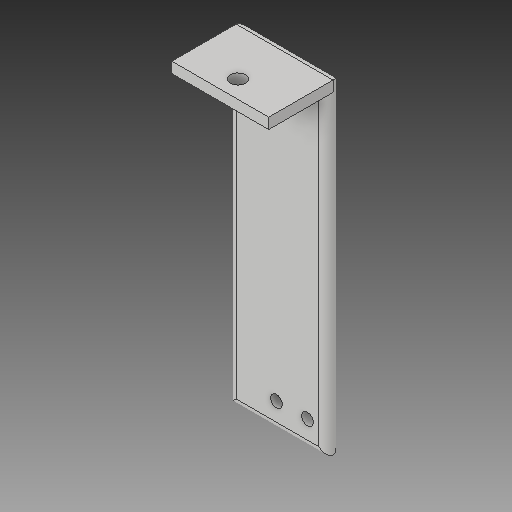
# Autodesk Inventor part: Chain_fixture
Saved by Autodesk Inventor 2019.3 (Build 233278000, 278)
## iProperties
Created: 2020-09-10
Part Number: Chain_fixture
Material: Generisch
Document SubType Name: Modeling
Designer: Nicolas Frick
Density: 1 g/cm^3
Appearance: Vorgabe
Author: Nicolas Frick
Autodesk Inventor part; units mm, degrees
ref_plane "YZ Plane" through (0, 0, 0) normal (1, 0, 0) x (0, 1, 0)
ref_plane "XZ Plane" through (0, 0, 0) normal (0, 1, 0) x (-1, 0, 0)
ref_plane "XY Plane" through (0, 0, 0) normal (0, 0, 1) x (1, 0, 0)
sketch "Skizze1" plane through (0, 0, 0) normal (0, 0, 1) x (1, 0, 0)
  line L0 (10, 15) -> (45.7133, 15) construction
  line L1 (10, 15) -> (10, -10) construction
  line L2 (37.1394, -10) -> (10, -10) construction
  line L3 (37.1394, -10) -> (37.1394, 14.1) construction
  line L4 (37.1394, 14.1) -> (45.7133, 14.1) construction
  line L5 (45.7133, 14.1) -> (45.7133, 15) construction
  line L6 (10, -10) -> (37.1394, -10)
  line L7 (37.1394, -10) -> (37.1394, 59.9176)
  line L8 (37.1394, 59.9176) -> (10, 59.9176)
  line L9 (10, 59.9176) -> (10, -10)
  point P0 (0, 0)
  constraints: 8 end point, 2 parallel, 1 horizontal, 1 perpendicular
extrude "Extrusion1" add sketch "Skizze1" along normal blind 4
sketch "Skizze2" plane through (0, 0, 0) normal (0, 0, -1) x (-1, 0, 0)
  line L0 (-37.1394, 59.9176) -> (-10, 59.9176) projected
  line L1 (-10, 59.9176) -> (-37.1394, 59.9176)
  line L2 (-37.1394, 59.9176) -> (-37.1394, 62.9176)
  line L3 (-37.1394, 62.9176) -> (-10, 62.9176)
  line L4 (-10, 62.9176) -> (-10, 59.9176)
  point P0 (0, 0)
  dimension "d2" = 3
  constraints: 8 end point, 2 parallel, 1 horizontal, 1 perpendicular
  measures "d2" distance of L1.end L2.end
extrude "Extrusion2" add sketch "Skizze2" against normal blind 20
sketch "Skizze4" plane through (10, 62.9176, 0) normal (0, 1, 0) x (1, 0, 0)
  line L0 (27.1394, -4) -> (27.1394, -73.6709) construction
  line L1 (-71.0464, -73.5081) -> (53.1741, -73.5081) construction
  line L2 (53.1741, -72.4315) -> (53.1741, -73.5081) construction
  arc A0 (58.1741, -67.4315) -> (53.1741, -72.4315) centre (58.1741, -72.4315) ccw construction
  line L3 (62.2394, -67.4315) -> (58.1741, -67.4315) construction
  line L4 (62.2394, -59.1955) -> (62.2394, -67.4315) construction
  arc A1 (65.5394, -59.1955) -> (62.2394, -59.1955) centre (63.8894, -59.1955) ccw construction
  line L5 (65.5394, -67.4315) -> (65.5394, -59.1955) construction
  line L6 (81.2394, -67.4315) -> (65.5394, -67.4315) construction
  arc A2 (76.4341, -48.82) -> (81.2394, -67.4315) centre (125.2788, -46.1349) ccw construction
  arc A3 (76.4267, -48.4999) -> (76.4341, -48.82) centre (81.4265, -48.5455) ccw construction
  arc A4 (76.4267, -48.4999) -> (35.4184, -9) centre (29.7163, -55.9569) ccw construction
  line L7 (35.4184, -9) -> (-5, -9) construction
  line L8 (-5, -9) -> (-5, 9.9226) construction
  line L9 (-5, 9.9226) -> (-10, 9.9226) construction
  line L10 (-10, 9.9226) -> (-10, 9.9096) construction
  line L11 (-10, 9.9096) -> (-37.7867, 9.9096) construction
  arc A5 (-37.7867, 9.9096) -> (-54.9732, -24.6463) centre (-14.5965, -23.176) ccw construction
  arc A6 (-54.9732, -24.6463) -> (-71.0464, -73.5081) centre (23.4557, -77.5201) ccw construction
  arc A7 (-40.4634, -62.3724) -> (-28.4634, -62.3724) centre (-34.4634, -62.3724) ccw construction
  line L12 (-40.4634, -62.3724) -> (-40.4634, -47.5724) construction
  arc A8 (-28.4634, -47.5724) -> (-40.4634, -47.5724) centre (-34.4634, -47.5724) ccw construction
  line L13 (-28.4634, -47.5724) -> (-28.4634, -62.3724) construction
  arc A9 (-40.4634, -16.9802) -> (-28.4634, -16.9802) centre (-34.4634, -16.9802) ccw construction
  line L14 (-40.4634, -16.9802) -> (-40.4634, -2.1802) construction
  arc A10 (-28.4634, -2.1802) -> (-40.4634, -2.1802) centre (-34.4634, -2.1802) ccw construction
  line L15 (-28.4634, -2.1802) -> (-28.4634, -16.9802) construction
  line L16 (37.2394, -63.0832) -> (59.5394, -63.0832) construction
  line L17 (37.2394, -34.3078) -> (37.2394, -63.0832) construction
  arc A11 (59.5394, -34.3078) -> (37.2394, -34.3078) centre (48.3894, -34.3078) ccw construction
  line L18 (59.5394, -63.0832) -> (59.5394, -34.3078) construction
  arc A12 (62.2394, -38.1955) -> (65.5394, -38.1955) centre (63.8894, -38.1955) ccw construction
  line L19 (62.2394, -28.1955) -> (62.2394, -38.1955) construction
  arc A13 (65.5394, -28.1955) -> (62.2394, -28.1955) centre (63.8894, -28.1955) ccw construction
  line L20 (65.5394, -38.1955) -> (65.5394, -28.1955) construction
  arc A14 (34.5394, -59.1955) -> (31.2394, -59.1955) centre (32.8894, -59.1955) ccw construction
  line L21 (34.5394, -67.4315) -> (34.5394, -59.1955) construction
  line L22 (31.2394, -67.4315) -> (34.5394, -67.4315) construction
  line L23 (31.2394, -59.1955) -> (31.2394, -67.4315) construction
  arc A15 (31.2394, -38.1955) -> (34.5394, -38.1955) centre (32.8894, -38.1955) ccw construction
  line L24 (31.2394, -28.1955) -> (31.2394, -38.1955) construction
  arc A16 (34.5394, -28.1955) -> (31.2394, -28.1955) centre (32.8894, -28.1955) ccw construction
  line L25 (34.5394, -38.1955) -> (34.5394, -28.1955) construction
  line L26 (0, -4) -> (0, -78.5081) construction
  line L27 (27.1394, -20) -> (0, -20) construction
  circle A17 centre (13.5697, -15.0495) radius 2.1
  point P0 (-10, 0)
  dimension "d11" = 4.2
  constraints: 1 centre point
  measures "d11" diameter of A17
extrude "Extrusion4" cut sketch "Skizze4" against normal through all
sketch "Skizze5" plane through (10, -10, 0) normal (0, -1, 0) x (1, 0, 0)
  line L0 (0, 0) -> (27.1394, 0) projected
  line L1 (27.1394, 0) -> (27.1394, 4) projected
  line L2 (0, 4) -> (27.1394, 4) projected
  line L3 (0, 0) -> (0, 4) projected
  point P0 (-10, 0)
extrude "Extrusion5" add sketch "Skizze5" along normal blind 18
sketch "Skizze6" plane through (0, 0, 0) normal (0, 0, -1) x (-1, 0, 0)
  arc A0 (-23.2894, -22.5324) -> (-23.2894, -19.2324) centre (-23.2894, -20.8824) ccw construction
  arc A1 (-31.9894, -19.2324) -> (-31.9894, -22.5324) centre (-31.9894, -20.8824) ccw construction
  circle A2 centre (-31.9894, -20.8824) radius 1.65
  circle A3 centre (-23.2894, -20.8824) radius 1.65
  point P0 (0, 0)
  constraints: 2 centre point, 2 coincident, 2 concentric
extrude "Extrusion6" cut sketch "Skizze6" against normal through all
fillet "Rundung3" radius 2 7 edges at (37.1394, 17.4588, 0) (23.5697, -28, 0) (10, 17.4588, 0) (37.1394, 15.9588, 4) (23.5697, -28, 4) (23.5697, 62.9176, 0) (10, 15.9588, 4)
